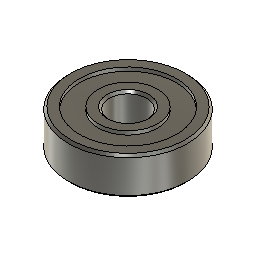
2022-07-06_clankite-v4 (Autodesk Fusion 360 archive; units mm, degrees)
design "PP_BRNG_625-5x16x5"
Autodesk Fusion 360 part; units mm, degrees
sketch "Sketch1" plane through (0, 0, 0) normal (0, 1, 0) x (1, 0, 0)
  line L0 (2.5, -2.5) -> (4, -2.5)
  line L1 (4, 2.5) -> (2.5, 2.5)
  line L2 (2.5, 2.5) -> (2.5, -2.5)
  line L3 (6.5, -2.5) -> (8, -2.5)
  line L4 (8, -2.5) -> (8, 2.5)
  line L5 (8, 2.5) -> (6.5, 2.5)
  line L6 (4, -2) -> (6.5, -2)
  line L7 (4, 2) -> (6.5, 2)
  line L8 (4, -2.5) -> (4, -2)
  line L9 (4, 2) -> (4, 2.5)
  line L10 (6.5, 2.5) -> (6.5, 2)
  line L11 (6.5, -2) -> (6.5, -2.5)
  line L12 (8, 0) -> (0, 0) construction
  point P0 (2.5, 0)
  dimension "d1" = 2.5
  dimension "d2" = 8
  dimension "d4" = 0.5
  dimension "d5" = 5
  dimension "d8" = 1.5
  constraint horizontal L0
  constraint vertical L8
  constraint horizontal L1
  constraint vertical L2
  constraint horizontal L3
  constraint vertical L4
  constraint horizontal L5
  constraint vertical L10
  constraint coincident L6.end L10
  constraint perpendicular L6 L10
  constraint coincident L7.start L8
  constraint perpendicular L7 L8
  constraint collinear L8 L9
  constraint collinear L10 L11
  constraint midpoint L4 L12.start
  constraint coincident L12.end origin
  constraint horizontal L12
  constraint midpoint L2 P0
  constraint coincident L12 P0
  constraint equal L0 L3
  constraint equal L8 L9
  constraint coincident L0 L3.start
  measures "d1" distance of L12.end L2
  measures "d2" distance of L12.end L4
  measures "d4" distance of L0.end L6.start
  measures "d5" distance of L3.end L4.end
  measures "d8" distance of L0.start L0.end
revolve "Revolve1" add sketch "Sketch1" angle 360 about axis through (0, 0, 1.75) along (0, 0, 1)
chamfer "Chamfer1" distance 0.3 angle 45 4 edges at (-2.3308, -0.904, 2.5) (-7.4586, -2.8929, 2.5) (-7.4586, -2.8929, -2.5) (-2.3308, -0.904, -2.5)
equation "d1 = ( 5 / 2 ) * 1 mm"
equation "d2 = ( 16 / 2 ) * 1 mm"

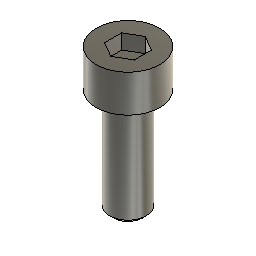
design "HW_M5x14-SHCS"
Autodesk Fusion 360 part; units mm, degrees
sketch "Sketch1" plane through (0, 0, 0) normal (0, 1, 0) x (1, 0, 0)
  line L0 (0, -5) -> (0, 14)
  line L1 (0, 14) -> (1.95, 14)
  line L2 (1.95, 14) -> (2.45, 13.5)
  line L3 (2.45, 13.5) -> (2.45, 0)
  line L4 (2.45, 0) -> (4.25, 0)
  line L5 (4.25, 0) -> (4.25, -5)
  line L6 (4.25, -5) -> (0, -5)
  dimension "d1" = 14
  dimension "d2" = 45
  dimension "d3" = 0.5
  dimension "d4" = 2.45
  dimension "d5" = 5
  dimension "d6" = 4.25
  constraint vertical L0
  constraint perpendicular L0 L1
  constraint perpendicular L1 L3
  constraint perpendicular L3 L4
  constraint perpendicular L4 L5
  constraint horizontal L6
  constraint coincident origin L0
  constraint coincident origin L4
  measures "d1" distance of origin L1
  measures "d2" angle of L1 L2
  measures "d3" horizontal distance of L1.end L2.end
  measures "d4" distance of L0.end L3
  measures "d5" distance of L4.end L5.end
  measures "d6" distance of L0.start L5.end
revolve "Revolve1" add sketch "Sketch1" angle 360 about axis through (0, 0, 5) along (0, 0, -1)
sketch "Sketch2" plane through (0, 0, 5) normal (0, 0, 1) x (-1, 0, 0)
  circle A0 centre (0, 0) radius 4.25
  line L0 (-2, -1.1547) -> (0, -2.3094)
  line L1 (0, -2.3094) -> (2, -1.1547)
  line L2 (2, -1.1547) -> (2, 1.1547)
  line L3 (2, 1.1547) -> (0, 2.3094)
  line L4 (0, 2.3094) -> (-2, 1.1547)
  line L5 (-2, 1.1547) -> (-2, -1.1547)
  dimension "d8" = 4
  constraint coincident A0.centre origin
  constraint vertical L5
  measures "d8" distance of L1.end L5
extrude "Extrude1" cut sketch "Sketch2" against normal blind 2 contours L0 L1 L2 L3 L4 L5
equation "d4 = ( 4.9 / 2 ) * 1 mm"
equation "d6 = ( 8.5 / 2 ) * 1 mm"

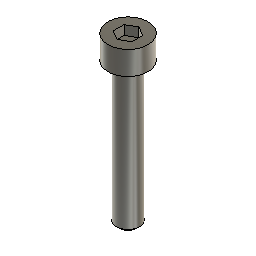
design "HW_M5x30-SHCS"
Autodesk Fusion 360 part; units mm, degrees
sketch "Sketch1" plane through (0, 0, 0) normal (0, 1, 0) x (1, 0, 0)
  line L0 (0, -5) -> (0, 30)
  line L1 (0, 30) -> (1.95, 30)
  line L2 (1.95, 30) -> (2.45, 29.5)
  line L3 (2.45, 29.5) -> (2.45, 0)
  line L4 (2.45, 0) -> (4.25, 0)
  line L5 (4.25, 0) -> (4.25, -5)
  line L6 (4.25, -5) -> (0, -5)
  dimension "d1" = 30
  dimension "d2" = 45
  dimension "d3" = 0.5
  dimension "d4" = 2.45
  dimension "d5" = 5
  dimension "d6" = 4.25
  constraint vertical L0
  constraint perpendicular L0 L1
  constraint perpendicular L1 L3
  constraint perpendicular L3 L4
  constraint perpendicular L4 L5
  constraint horizontal L6
  constraint coincident origin L0
  constraint coincident origin L4
  measures "d1" distance of origin L1
  measures "d2" angle of L1 L2
  measures "d3" horizontal distance of L1.end L2.end
  measures "d4" distance of L0.end L3
  measures "d5" distance of L4.end L5.end
  measures "d6" distance of L0.start L5.end
revolve "Revolve1" add sketch "Sketch1" angle 360 about axis through (0, 0, 5) along (0, 0, -1)
sketch "Sketch2" plane through (0, 0, 5) normal (0, 0, 1) x (-1, 0, 0)
  circle A0 centre (0, 0) radius 4.25
  line L0 (-2, -1.1547) -> (0, -2.3094)
  line L1 (0, -2.3094) -> (2, -1.1547)
  line L2 (2, -1.1547) -> (2, 1.1547)
  line L3 (2, 1.1547) -> (0, 2.3094)
  line L4 (0, 2.3094) -> (-2, 1.1547)
  line L5 (-2, 1.1547) -> (-2, -1.1547)
  dimension "d8" = 4
  constraint coincident A0.centre origin
  constraint vertical L5
  measures "d8" distance of L1.end L5
extrude "Extrude1" cut sketch "Sketch2" against normal blind 2 contours L0 L1 L2 L3 L4 L5
equation "d4 = ( 4.9 / 2 ) * 1 mm"
equation "d6 = ( 8.5 / 2 ) * 1 mm"

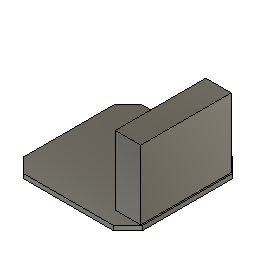
design "Fab Step"
Autodesk Fusion 360 part; units mm, degrees
sketch "Sketch1" plane through (0, 0, 0) normal (0, 0, 1) x (1, 0, 0)
  line L0 (21, 21) -> (-21, 21)
  line L1 (-21, 21) -> (-21, -21)
  line L2 (-21, -21) -> (21, -21)
  line L3 (21, -21) -> (21, 21)
  line L4 (21, 21) -> (-21, -21) construction
  line L5 (-21, 21) -> (21, -21) construction
  line L6 (-15.5, 15.5) -> (15.5, 15.5) construction
  line L7 (15.5, 15.5) -> (15.5, -15.5) construction
  line L8 (15.5, -15.5) -> (-15.5, -15.5) construction
  line L9 (-15.5, -15.5) -> (-15.5, 15.5) construction
  circle A0 centre (-15.5, 15.5) radius 1.5
  circle A1 centre (-15.5, -15.5) radius 1.5
  circle A2 centre (15.5, -15.5) radius 1.5
  circle A3 centre (15.5, 15.5) radius 1.5
  circle A4 centre (0, 0) radius 2.5
  line L10 (21, -16) -> (11.5, -16)
  line L11 (11.5, -16) -> (11.5, 16)
  line L12 (11.5, 16) -> (21, 16)
  line L13 (11.5, 0) -> (0, 0) construction
  line L14 (20.5, -16) -> (20.5, 16)
  dimension "d1" = 42
  dimension "d3" = 31
  dimension "d4" = 3
  dimension "d5" = 5
  dimension "d18" = 32
  dimension "d19" = 0.5
  dimension "d24" = 9
  constraint perpendicular L0 L1
  constraint parallel L0 L2
  constraint parallel L1 L3
  constraint horizontal L0
  constraint coincident L4 A4.centre
  constraint coincident L5 A4.centre
  constraint coincident A4.centre L13.end
  constraint equal L0 L1
  constraint horizontal L6
  constraint vertical L7
  constraint horizontal L8
  constraint vertical L9
  constraint coincident L5 L7.end
  constraint coincident L5 L6.start
  constraint coincident L4 L6.end
  constraint coincident L6.start L9.end
  constraint coincident L8.end L9.start
  constraint coincident L7.end L8.start
  constraint coincident L6.end L7.start
  constraint equal A0 A3
  constraint equal A0 A1
  constraint equal A0 A2
  constraint coincident L3 L10.start
  constraint perpendicular L3 L10
  constraint perpendicular L10 L11
  constraint coincident L3 L12.end
  constraint perpendicular L3 L12
  constraint midpoint L11 L13.start
  constraint horizontal L13
  constraint coincident L10 L14.start
  constraint coincident L12 L14.end
  constraint perpendicular L12 L14
  measures "d1" distance of L0.start L0.end
  measures "d3" distance of L6.start L6.end
  measures "d4" diameter of A0
  measures "d5" diameter of A4
  measures "d18" distance of L10.end L11.end
  measures "d19" distance of L3 L14
  measures "d24" distance of L11 L14
extrude "Extrude5" add sketch "Sketch1" along normal blind 1.6 contours L0 L1 L2 L3 A2 A3 L10 L11 L12 | L3 L10 L12 L14 | A2 A3 L10 L11 L12 L14 | A3 L12 | A3 L12 | A2 L10 | A2 L10 | A0 | A1 | A4
extrude "Extrude6" add sketch "Sketch1" along normal blind 24.4 from surface at 1.6 contours A2 A3 L10 L11 L12 L14 | A3 L12 | A2 L10 picked at (15.1098, 15.5207) picked at (15.6311, -15.3508)
chamfer "Chamfer2" distance 5 angle 45 4 edges at (21, -21, 0.8) (21, 21, 0.8) (-21, -21, 0.8) (-21, 21, 0.8)
